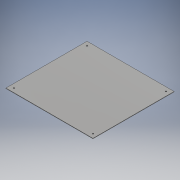
# Autodesk Inventor part: bundplade
Saved by Autodesk Inventor 2018 (Build 220112000, 112)
## iProperties
Created: 2018-01-29
Part Number: bundplade
Material: Steel
Document SubType Name: Modeling
Designer: MikkelS
Density: 7.85 g/cm^3
Appearance: Plate
Author: MikkelS
Autodesk Inventor part; units mm, degrees
ref_plane "YZ Plane" through (0, 0, 0) normal (1, 0, 0) x (0, 1, 0)
ref_plane "XZ Plane" through (0, 0, 0) normal (0, 1, 0) x (-1, 0, 0)
ref_plane "XY Plane" through (0, 0, 0) normal (0, 0, 1) x (1, 0, 0)
sketch "Sketch1" plane through (0, 0, 0) normal (0, 0, 1) x (1, 0, 0)
  line L0 (0, 0) -> (0, 383)
  line L1 (0, 383) -> (411, 383)
  line L2 (411, 383) -> (411, 0)
  line L3 (411, 0) -> (0, 0)
  dimension "d0" = 383
  dimension "d1" = 411
  constraints: 8 end point, 3 perpendicular, 1 vertical
  measures "d0" distance of L0.start L0.end
  measures "d1" distance of L0.end L1.end
extrude "Extrusion1" add sketch "Sketch1" along normal blind 2
sketch "Sketch2" plane through (0, 0, 2) normal (0, 0, 1) x (1, 0, 0)
  line L0 (0, 0) -> (0, 18.82)
  line L1 (0, 383) -> (0, 0) projected
  line L2 (0, 18.82) -> (19, 18.82)
  circle A0 centre (19, 18.82) radius 3
  dimension "d4" = 18.82
  dimension "d5" = 19
  dimension "d6" = 6
  constraints: 4 end point, 1 centre point, 1 coincident, 1 horizontal, 1 point on line
  measures "d4" distance of L0.start L0.end
  measures "d5" distance of L0.end L2.end
  measures "d6" diameter of A0
hole "Hole1" at (19, 18.82, 2) direction (0, 0, -1) diameter 6 end through all
sketch "Sketch3" plane through (0, 0, 2) normal (0, 0, 1) x (1, 0, 0)
  line L0 (411, 0) -> (0, 0) projected
  line L1 (411, 0) -> (411, 18.82)
  line L2 (411, 383) -> (411, 0) projected
  line L3 (411, 18.82) -> (392, 18.82)
  circle A0 centre (392, 18.82) radius 3
  dimension "d14" = 18.82
  dimension "d15" = 19
  dimension "d16" = 6
  constraints: 4 end point, 1 centre point, 1 coincident, 1 perpendicular, 1 point on line
  measures "d14" distance of L0.start L1.end
  measures "d15" distance of L1.end L3.end
  measures "d16" diameter of A0
hole "Hole2" at (392, 18.82, 2) direction (0, 0, -1) diameter 6 end through all
sketch "Sketch4" plane through (0, 0, 2) normal (0, 0, 1) x (1, 0, 0)
  line L0 (0, 382.7342) -> (0, 363.9142)
  line L1 (0, 0) -> (0, 383) projected
  line L2 (0, 363.9142) -> (19, 363.9142)
  circle A0 centre (19, 363.9142) radius 3
  dimension "d24" = 18.82
  dimension "d25" = 19
  dimension "d26" = 6
  constraints: 4 end point, 1 centre point, 1 coincident, 1 perpendicular, 1 point on line
  measures "d24" distance of L0.start L0.end
  measures "d25" distance of L0.end L2.end
  measures "d26" diameter of A0
hole "Hole3" at (19, 363.9142, 2) direction (0, 0, -1) diameter 6 end through all
sketch "Sketch5" plane through (0, 0, 2) normal (0, 0, 1) x (1, 0, 0)
  line L0 (411, 383) -> (411, 0) projected
  line L1 (411, 383) -> (411, 364.18)
  line L2 (411, 364.18) -> (392, 364.18)
  circle A0 centre (392, 364.18) radius 3
  point P0 (0, 0)
  dimension "d34" = 18.82
  dimension "d35" = 19
  dimension "d36" = 6
  constraints: 4 end point, 1 centre point, 1 coincident, 1 perpendicular, 1 point on line
  measures "d34" distance of L0.start L1.end
  measures "d35" distance of L1.end L2.end
  measures "d36" diameter of A0
hole "Hole4" at (392, 364.18, 2) direction (0, 0, -1) diameter 6 end through all
body "Solid1"
